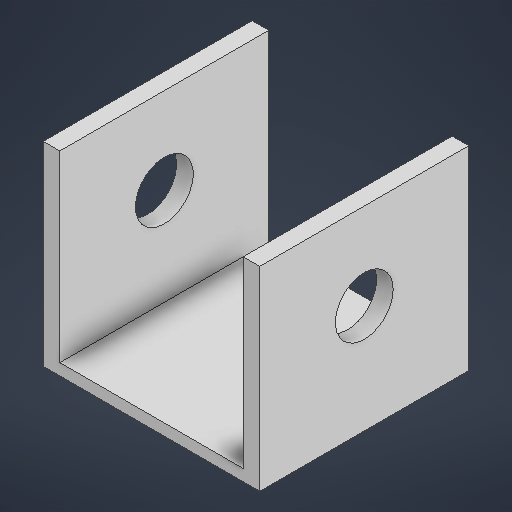
# Autodesk Inventor part: Rough_1in_U_Bracket
Saved by Autodesk Inventor 2026.1 (Build 301233000, 233)
## iProperties
Created: 2026-09-15
Part Number: Rough_1in_U_Bracket
Material: Generic
Document SubType Name: Modeling
Designer: share
Density: 1 g/cm^3
Appearance: Default
Author: share
Autodesk Inventor part; units mm, degrees
ref_plane "YZ Plane" through (0, 0, 0) normal (1, 0, 0) x (0, 1, 0)
ref_plane "XZ Plane" through (0, 0, 0) normal (0, 1, 0) x (-1, 0, 0)
ref_plane "XY Plane" through (0, 0, 0) normal (0, 0, 1) x (1, 0, 0)
sketch "Sketch1" plane through (0, 0, 0) normal (0, 1, 0) x (-1, 0, 0)
  line L0 (-15, -14.4762) -> (15, -14.4762)
  line L1 (15, -14.4762) -> (15, 14.4762)
  line L2 (15, 14.4762) -> (-15, 14.4762)
  line L3 (-15, 14.4762) -> (-15, -14.4762)
  line L4 (-15, -14.4762) -> (15, 14.4762) construction
  line L5 (15, -14.4762) -> (-15, 14.4762) construction
  point P0 (0, 0)
  dimension "d0" = 30
  constraints: 12 end point, 2 midpoint, 2 parallel, 1 horizontal, 1 perpendicular
  measures "d0" distance between parallel lines of L3 L1
extrude "Extrusion1" add sketch "Sketch1" along normal blind 1.5875
sketch "Sketch2" plane through (0, 1.5875, 0) normal (0, 1, 0) x (1, 0, 0)
  line L0 (-15, 14.4762) -> (-15, -14.4762) projected
  line L1 (-15, -14.4762) -> (15, -14.4762) projected
  line L2 (15, -14.4762) -> (15, 14.4762) projected
  line L3 (15, 14.4762) -> (-15, 14.4762) projected
  line L4 (-12.7, -14.4762) -> (-12.7, 14.4762)
  line L5 (0, 20.2667) -> (0, -20.2667) projected
  line L6 (12.7, -14.4762) -> (12.7, 14.4762)
  point P0 (0, 0)
  dimension "d3" = 25.4
  constraints: 4 end point, 2 point on line, 2 symmetric about line, 1 perpendicular
  measures "d3" distance between parallel lines of L6 L4
extrude "Extrusion2" add sketch "Sketch2" along normal blind 25.4 contours L3 L4 L1 L0 | L3 L2 L1 L6
sketch "Sketch3" plane through (15, 0, 14.4762) normal (1, 0, 0) x (0, 0, -1)
  line L0 (-5.7905, 0) -> (34.7429, 0) construction
  line L1 (14.4762, -5.3975) -> (14.4762, 32.385) construction
  point P0 (14.4762, 0)
  point P1 (14.4762, 15)
  dimension "d6" = 15
  constraints: 1 point on line
  measures "d6" distance from line of L0 point (14.476, 15)
hole "Hole1" at (15, 15, 0) direction (-1, 0, 0) diameter 8 end through all
body "Solid1"
